Autodesk Fusion 360 part; units mm, degrees
note: some values were not read from the file. Chosen so that the rebuilt part matches the saved one: a side. Set by a fixed rule: which sketch regions a step uses.
(part 2 of 2)
sketch "Sketch13" plane through (0, 0, 19.74) normal (0, 0, -1) x (-1, 0, 0)
  line L0 (59.2047, 4.6574) -> (48.6047, 15.1574)
  line L1 (48.6047, -14.8158) -> (59.2047, -4.3158)
  arc A0 (-51.6422, 17.0699) -> (-55.1422, 13.5699) centre (-51.6422, 13.5699) ccw
  arc A1 (35.5416, -3.8292) -> (37.5416, -1.8292) centre (35.5416, -1.8292) ccw
  line L2 (47.9916, -8.3292) -> (47.9916, -12.3292)
  arc A2 (46.1416, -3.6792) -> (47.9916, -1.8292) centre (46.1416, -1.8292) ccw
  arc A3 (-47.6422, 7.7199) -> (-45.7922, 9.5699) centre (-47.6422, 9.5699) ccw
  line L3 (52.7416, 4.0208) -> (56.7416, 4.0208)
  line L4 (40.2916, -12.3292) -> (40.2916, -8.3292)
  line L5 (40.2916, -1.8292) -> (40.2916, 2.1708)
  arc A4 (-45.6422, -7.4301) -> (-47.6422, -5.4301) centre (-47.6422, -7.4301) ccw
  line L6 (39.6785, 15.1574) -> (29.0785, 4.6574)
  line L7 (58.5916, 2.1708) -> (58.5916, -1.8292)
  line L8 (40.2916, 8.6708) -> (40.2916, 12.6708)
  arc A5 (-47.6422, 7.5699) -> (-45.6422, 9.5699) centre (-47.6422, 9.5699) ccw
  arc A6 (46.1416, 6.8208) -> (47.9916, 8.6708) centre (46.1416, 8.6708) ccw
  line L9 (46.1416, 16.1708) -> (42.1416, 16.1708)
  arc A7 (42.1416, -6.4792) -> (40.2916, -8.3292) centre (42.1416, -8.3292) ccw
  line L10 (37.3916, 2.1708) -> (37.3916, -1.8292)
  arc A8 (42.1416, 4.0208) -> (40.2916, 2.1708) centre (42.1416, 2.1708) ccw
  arc A9 (-51.6422, -5.4301) -> (-53.6422, -7.4301) centre (-51.6422, -7.4301) ccw
  arc A10 (40.2916, 8.6708) -> (42.1416, 6.8208) centre (42.1416, 8.6708) ccw
  line L11 (46.1416, -15.8292) -> (48.451, -15.8292) construction
  line L12 (50.8916, -1.8292) -> (50.8916, 2.1708)
  arc A11 (29.5416, -1.8292) -> (31.5416, -3.8292) centre (31.5416, -1.8292) ccw
  line L13 (-45.6422, -7.4301) -> (-45.6422, -11.4301)
  line L14 (42.1416, -6.4792) -> (46.1416, -6.4792)
  arc A12 (60.2416, 2.1708) -> (56.7416, 5.6708) centre (56.7416, 2.1708) ccw
  arc A13 (37.5416, 2.1708) -> (35.5416, 4.1708) centre (35.5416, 2.1708) ccw
  arc A14 (58.5916, 2.1708) -> (56.7416, 4.0208) centre (56.7416, 2.1708) ccw
  line L15 (-45.6422, 13.5699) -> (-45.6422, 9.5699)
  arc A15 (42.1416, 14.5208) -> (40.2916, 12.6708) centre (42.1416, 12.6708) ccw
  arc A16 (50.8916, -1.8292) -> (52.7416, -3.6792) centre (52.7416, -1.8292) ccw
  line L16 (42.1416, 14.5208) -> (46.1416, 14.5208)
  line L17 (-47.6422, -13.4301) -> (-51.6422, -13.4301)
  arc A17 (40.2916, -1.8292) -> (42.1416, -3.6792) centre (42.1416, -1.8292) ccw
  line L18 (-47.6422, 7.5699) -> (-51.6422, 7.5699)
  line L19 (28.0416, 2.1708) -> (28.0416, -1.8292)
  line L20 (31.5416, 4.0208) -> (35.5416, 4.0208)
  line L21 (47.9916, 12.6708) -> (47.9916, 8.6708)
  line L22 (42.1416, 4.0208) -> (46.1416, 4.0208)
  line L23 (-53.6422, 9.5699) -> (-53.6422, 13.5699)
  arc A18 (47.9916, 2.1708) -> (46.1416, 4.0208) centre (46.1416, 2.1708) ccw
  arc A19 (49.6416, 12.6708) -> (46.1416, 16.1708) centre (46.1416, 12.6708) ccw
  line L24 (-51.6422, 15.5699) -> (-47.6422, 15.5699)
  arc A20 (28.0416, -1.8292) -> (31.5416, -5.3292) centre (31.5416, -1.8292) ccw
  line L25 (47.9916, 2.1708) -> (47.9916, -1.8292)
  arc A21 (46.1416, -15.8292) -> (49.6416, -12.3292) centre (46.1416, -12.3292) ccw
  arc A22 (52.7416, 4.0208) -> (50.8916, 2.1708) centre (52.7416, 2.1708) ccw
  arc A23 (-51.6422, 15.5699) -> (-53.6422, 13.5699) centre (-51.6422, 13.5699) ccw
  line L26 (46.1416, -3.6792) -> (42.1416, -3.6792)
  line L27 (-53.6422, -11.4301) -> (-53.6422, -7.4301)
  line L28 (56.7416, -3.6792) -> (52.7416, -3.6792)
  arc A24 (-45.7922, 13.5699) -> (-47.6422, 15.4199) centre (-47.6422, 13.5699) ccw
  arc A25 (-47.6422, -13.2801) -> (-45.7922, -11.4301) centre (-47.6422, -11.4301) ccw
  line L29 (29.0785, -4.3158) -> (39.6785, -14.8158)
  arc A26 (29.6916, -1.8292) -> (31.5416, -3.6792) centre (31.5416, -1.8292) ccw
  arc A27 (40.2916, -12.3292) -> (42.1416, -14.1792) centre (42.1416, -12.3292) ccw
  arc A28 (-44.1422, 13.5699) -> (-47.6422, 17.0699) centre (-47.6422, 13.5699) ccw
  arc A29 (38.6416, -12.3292) -> (42.1416, -15.8292) centre (42.1416, -12.3292) ccw
  line L30 (-45.7922, 13.5699) -> (-45.7922, 9.5699)
  line L31 (44.1416, -14.6745) -> (42.1416, -15.8292)
  line L32 (-51.6422, 17.0699) -> (-47.6422, 17.0699)
  line L33 (46.1416, -14.1792) -> (42.1416, -14.1792)
  arc A30 (-51.6422, -5.5801) -> (-53.4922, -7.4301) centre (-51.6422, -7.4301) ccw
  arc A31 (56.7416, -5.3292) -> (60.2416, -1.8292) centre (56.7416, -1.8292) ccw
  arc A32 (-51.6422, 15.4199) -> (-53.4922, 13.5699) centre (-51.6422, 13.5699) ccw
  line L34 (-55.1422, -11.4301) -> (-55.1422, 13.5699)
  line L35 (29.5416, -1.8292) -> (29.5416, 2.1708)
  arc A33 (31.5416, 4.0208) -> (29.6916, 2.1708) centre (31.5416, 2.1708) ccw
  arc A34 (-53.4922, -11.4301) -> (-51.6422, -13.2801) centre (-51.6422, -11.4301) ccw
  arc A35 (-53.4922, 9.5699) -> (-51.6422, 7.7199) centre (-51.6422, 9.5699) ccw
  line L36 (-47.6422, -14.9301) -> (-51.6422, -14.9301)
  line L37 (-53.4922, 9.5699) -> (-53.4922, 13.5699)
  line L38 (-44.1422, -11.4301) -> (-44.1422, 13.5699)
  line L39 (31.5416, 4.1708) -> (35.5416, 4.1708)
  arc A36 (-45.7922, -7.4301) -> (-47.6422, -5.5801) centre (-47.6422, -7.4301) ccw
  arc A37 (-47.6422, -14.9301) -> (-44.1422, -11.4301) centre (-47.6422, -11.4301) ccw
  arc A38 (35.5416, -3.6792) -> (37.3916, -1.8292) centre (35.5416, -1.8292) ccw
  line L40 (-45.7922, -7.4301) -> (-45.7922, -11.4301)
  line L41 (-51.6422, -5.5801) -> (-47.6422, -5.5801)
  line L42 (35.5416, -3.8292) -> (31.5416, -3.8292)
  line L43 (-47.6422, 7.7199) -> (-51.6422, 7.7199)
  line L44 (46.1416, -15.8292) -> (44.1416, -14.6745)
  arc A39 (47.9916, -8.3292) -> (46.1416, -6.4792) centre (46.1416, -8.3292) ccw
  arc A40 (31.5416, 5.6708) -> (28.0416, 2.1708) centre (31.5416, 2.1708) ccw
  line L45 (35.5416, -3.6792) -> (31.5416, -3.6792)
  line L46 (37.5416, 2.1708) -> (37.5416, -1.8292)
  arc A41 (56.7416, -3.6792) -> (58.5916, -1.8292) centre (56.7416, -1.8292) ccw
  line L47 (42.1416, -15.8292) -> (45.0396, -15.8292) construction
  arc A42 (-55.1422, -11.4301) -> (-51.6422, -14.9301) centre (-51.6422, -11.4301) ccw
  line L48 (42.1416, -15.8292) -> (46.1416, -15.8292)
  line L49 (-47.6422, -13.2801) -> (-51.6422, -13.2801)
  arc A43 (42.1416, 16.1708) -> (38.6416, 12.6708) centre (42.1416, 12.6708) ccw
  line L50 (46.1416, -3.8292) -> (42.1416, -3.8292)
  arc A44 (-45.6422, 13.5699) -> (-47.6422, 15.5699) centre (-47.6422, 13.5699) ccw
  line L51 (46.1416, 6.8208) -> (42.1416, 6.8208)
  line L52 (29.6916, -1.8292) -> (29.6916, 2.1708)
  arc A45 (46.1416, -14.1792) -> (47.9916, -12.3292) centre (46.1416, -12.3292) ccw
  line L53 (60.2416, -1.8292) -> (60.2416, 2.1708)
  line L54 (-51.6422, 15.4199) -> (-47.6422, 15.4199)
  line L55 (-53.4922, -11.4301) -> (-53.4922, -7.4301)
  arc A46 (37.3916, 2.1708) -> (35.5416, 4.0208) centre (35.5416, 2.1708) ccw
  arc A47 (31.5416, 4.1708) -> (29.5416, 2.1708) centre (31.5416, 2.1708) ccw
  arc A48 (-53.6422, -11.4301) -> (-51.6422, -13.4301) centre (-51.6422, -11.4301) ccw
  arc A49 (40.1416, -1.8292) -> (42.1416, -3.8292) centre (42.1416, -1.8292) ccw
  line L56 (46.1416, 6.6708) -> (42.1416, 6.6708)
  arc A50 (40.1416, -12.3292) -> (42.1416, -14.3292) centre (42.1416, -12.3292) ccw
  line L57 (48.1416, 2.1708) -> (48.1416, -1.8292)
  arc A51 (-53.6422, 9.5699) -> (-51.6422, 7.5699) centre (-51.6422, 9.5699) ccw
  arc A52 (46.1416, -3.8292) -> (48.1416, -1.8292) centre (46.1416, -1.8292) ccw
  line L58 (52.7416, 4.1708) -> (56.7416, 4.1708)
  arc A53 (40.1416, 8.6708) -> (42.1416, 6.6708) centre (42.1416, 8.6708) ccw
  arc A54 (42.1416, -6.3292) -> (40.1416, -8.3292) centre (42.1416, -8.3292) ccw
  arc A55 (47.9916, 12.6708) -> (46.1416, 14.5208) centre (46.1416, 12.6708) ccw
  arc A56 (56.7416, -3.8292) -> (58.7416, -1.8292) centre (56.7416, -1.8292) ccw
  line L59 (42.1416, -6.3292) -> (46.1416, -6.3292)
  line L60 (42.1416, 14.6708) -> (46.1416, 14.6708)
  line L61 (48.1416, 12.6708) -> (48.1416, 8.6708)
  arc A57 (58.7416, 2.1708) -> (56.7416, 4.1708) centre (56.7416, 2.1708) ccw
  line L62 (46.1416, -14.3292) -> (42.1416, -14.3292)
  line L63 (40.1416, -12.3292) -> (40.1416, -8.3292)
  arc A58 (42.1416, 14.6708) -> (40.1416, 12.6708) centre (42.1416, 12.6708) ccw
  line L64 (56.7416, -3.8292) -> (52.7416, -3.8292)
  arc A59 (-47.6422, -13.4301) -> (-45.6422, -11.4301) centre (-47.6422, -11.4301) ccw
  arc A60 (46.1416, -14.3292) -> (48.1416, -12.3292) centre (46.1416, -12.3292) ccw
  line L65 (50.7416, -1.8292) -> (50.7416, 2.1708)
  arc A61 (50.7416, -1.8292) -> (52.7416, -3.8292) centre (52.7416, -1.8292) ccw
  arc A62 (42.1416, 4.1708) -> (40.1416, 2.1708) centre (42.1416, 2.1708) ccw
  line L66 (40.1416, 8.6708) -> (40.1416, 12.6708)
  arc A63 (48.1416, -8.3292) -> (46.1416, -6.3292) centre (46.1416, -8.3292) ccw
  arc A64 (48.1416, 12.6708) -> (46.1416, 14.6708) centre (46.1416, 12.6708) ccw
  line L67 (48.1416, -8.3292) -> (48.1416, -12.3292)
  line L68 (40.1416, -1.8292) -> (40.1416, 2.1708)
  line L69 (42.1416, 4.1708) -> (46.1416, 4.1708)
  arc A65 (52.7416, 4.1708) -> (50.7416, 2.1708) centre (52.7416, 2.1708) ccw
  line L70 (-51.6422, -5.4301) -> (-47.6422, -5.4301)
  arc A66 (48.1416, 2.1708) -> (46.1416, 4.1708) centre (46.1416, 2.1708) ccw
  arc A67 (46.1416, 6.6708) -> (48.1416, 8.6708) centre (46.1416, 8.6708) ccw
  line L71 (58.7416, 2.1708) -> (58.7416, -1.8292)
  arc A68 (-47.6422, -2.9301) -> (-45.6422, -0.9301) centre (-47.6422, -0.9301) ccw
  arc A69 (-45.6422, 3.0699) -> (-47.6422, 5.0699) centre (-47.6422, 3.0699) ccw
  line L72 (-53.4922, -0.9301) -> (-53.4922, 3.0699)
  arc A70 (-47.6422, -2.7801) -> (-45.7922, -0.9301) centre (-47.6422, -0.9301) ccw
  line L73 (-45.7922, 3.0699) -> (-45.7922, -0.9301)
  line L74 (-45.6422, 3.0699) -> (-45.6422, -0.9301)
  line L75 (-51.6422, 5.0699) -> (-47.6422, 5.0699)
  arc A71 (-53.4922, -0.9301) -> (-51.6422, -2.7801) centre (-51.6422, -0.9301) ccw
  arc A72 (-51.6422, 4.9199) -> (-53.4922, 3.0699) centre (-51.6422, 3.0699) ccw
  line L76 (-47.6422, -2.9301) -> (-51.6422, -2.9301)
  arc A73 (-45.7922, 3.0699) -> (-47.6422, 4.9199) centre (-47.6422, 3.0699) ccw
  arc A74 (-51.6422, 5.0699) -> (-53.6422, 3.0699) centre (-51.6422, 3.0699) ccw
  line L77 (-47.6422, -2.7801) -> (-51.6422, -2.7801)
  line L78 (-51.6422, 4.9199) -> (-47.6422, 4.9199)
  line L79 (-53.6422, -0.9301) -> (-53.6422, 3.0699)
  arc A75 (-53.6422, -0.9301) -> (-51.6422, -2.9301) centre (-51.6422, -0.9301) ccw
  line L80 (-49.6422, -14.9301) -> (-49.6422, 17.0699) construction
  line L81 (-49.6422, -5.5801) -> (-49.6422, -4.1801) construction
  line L82 (-49.6422, 4.9199) -> (-49.6422, 6.3199) construction
  line L83 (-49.6422, 17.0699) -> (-49.6422, 16.2449) construction
  arc A76 (-55.1422, 8.8199) -> (-53.2922, 6.9699) centre (-53.2922, 8.8199) ccw
  arc A77 (-53.2922, -4.8301) -> (-55.1422, -6.6801) centre (-53.2922, -6.6801) ccw
  arc A78 (-53.2922, 5.6699) -> (-55.1422, 3.8199) centre (-53.2922, 3.8199) ccw
  arc A79 (-55.1422, -1.6801) -> (-53.2922, -3.5301) centre (-53.2922, -1.6801) ccw
  arc A80 (-49.6422, 5.6699) -> (-49.6422, 6.9699) centre (-49.6422, 6.3199) ccw
  line L84 (-49.6422, 6.9699) -> (-53.2922, 6.9699)
  line L85 (-53.2922, 5.6699) -> (-49.6422, 5.6699)
  arc A81 (-49.6422, -4.8301) -> (-49.6422, -3.5301) centre (-49.6422, -4.1801) ccw
  line L86 (-53.2922, -3.5301) -> (-49.6422, -3.5301)
  line L87 (-53.2922, -4.8301) -> (-49.6422, -4.8301)
  point P0 (42.95, -0.15)
  point P1 (0, -0.15)
  point P2 (-38.4431, -20.574)
  point P3 (-35.0431, -20.574)
  point P4 (23.3574, -20.574)
  point P5 (19.9574, -20.574)
  point P6 (-47.6422, -0.9301)
  point P7 (-51.6422, -0.9301)
  dimension "d137" = 0.15
  dimension "d138" = 0.15
  dimension "d139" = 0.15
  dimension "d140" = 0.15
  dimension "d141" = 0.15
  dimension "d142" = 0.15
  dimension "d144" = 0.15
  dimension "d145" = 1.5
  dimension "d146" = 1.5
  dimension "d147" = 1.5
  dimension "d148" = 1.5
  dimension "d149" = 1.5
  dimension "d150" = 1.5
  dimension "d151" = 1.5
  dimension "d152" = 1.5
  dimension "d153" = 1.5
  dimension "d154" = 1.5
  dimension "d155" = 150
  dimension "d156" = 0.15
  dimension "d185" = 1.4
  dimension "d186" = 1.4
  dimension "d190" = 0.825
  dimension "d193" = 0.65
  dimension "d194" = 0.65
  constraint coincident L1.start A21
  constraint coincident L1.end A31
  constraint tangent L1 A21
  constraint tangent L1 A31
  constraint coincident L0.start A12
  constraint coincident L0.end A19
  constraint coincident L6.start A43
  constraint coincident L6.end A40
  constraint coincident L29.start A20
  constraint coincident L29.end A29
  constraint tangent L0 A12
  constraint tangent L0 A19
  constraint tangent L6 A43
  constraint tangent L6 A40
  constraint tangent L29 A29
  constraint tangent A20 L29
  constraint tangent A21 L48
  constraint tangent A12 L53
  constraint tangent L9 A43
  constraint tangent L19 A20
  constraint tangent A0 L34
  constraint tangent A28 L38
  constraint horizontal L47
  constraint horizontal L11
  constraint midpoint L36 L80.start
  constraint midpoint L32 L80.end
  constraint perpendicular L32 L80
  constraint midpoint L41 L81.start
  constraint perpendicular L41 L81
  constraint midpoint L78 L82.start
  constraint perpendicular L75 L82
  constraint perpendicular L32 L83
  constraint coincident L80 A80.start
  constraint coincident L82.end A80.centre
  constraint tangent A76 L84
  constraint tangent A80 L85
  constraint coincident L80 A81.start
  constraint coincident L81.end A81.centre
  constraint tangent A81 L86
  constraint tangent A81 L87
  measures "d155" angle of L11 L44
  measures "d185" distance of L81.start L81.end
  measures "d186" distance of L82.start L82.end
  measures "d190" distance of L80.end L83.end
  measures "d193" radius of A80
  measures "d194" radius of A81
extrude "Extrude20" add sketch "Sketch13" along normal blind 0.2 separate body contours L0 L1 L6 L9 A12 L19 A19 A20 A21 L29 A29 L31 A31 L44 A40 A43 L53 | A0 A28 L32 L34 L36 L38 A37 A42 A76 A77 A78 A79 A80 L84 L85 A81 L86 L87 | A1 A11 A13 L35 L39 L42 L46 A47 | L2 L4 A7 L14 A27 L33 A39 A45 | A2 L5 A8 A17 L22 A18 L25 L26 | A3 A24 L30 A32 A35 L37 L43 L54 | L3 L7 L12 A14 A16 A22 L28 A41 | A4 A9 L13 L17 L27 A48 A59 L70 | L8 A6 A10 A15 L16 L21 L51 A55 | A5 L15 L18 L23 L24 A23 A44 A51 | L10 L20 A26 A33 A38 L45 L52 A46 | A25 A30 A34 A36 L40 L41 L49 L55 | L50 A49 L57 A52 A62 L68 L69 A66 | L56 A53 L60 L61 A58 L66 A64 A67 | A50 A54 L59 L62 L63 A60 A63 L67 | L58 A56 A57 L64 L65 A61 A65 L71 | A68 A69 L74 L75 L76 A74 L79 A75 | L72 A70 L73 A71 A72 A73 L77 L78 makes body 3 at (45.7739, 2.7408, 19.74) makes body 4 at (-50.6503, 1.7134, 19.74)
extrude "Extrude21" add sketch "Sketch13" against normal blind 4 contours L2 L4 A7 L14 A27 L33 A39 A45 | A2 L5 A8 A17 L22 A18 L25 L26 | A3 A24 L30 A32 A35 L37 L43 L54 | L3 L7 L12 A14 A16 A22 L28 A41 | L8 A6 A10 A15 L16 L21 L51 A55 | L10 L20 A26 A33 A38 L45 L52 A46 | A25 A30 A34 A36 L40 L41 L49 L55 | L72 A70 L73 A71 A72 A73 L77 L78 bodies 3 4
fillet "Fillet3" radius 1.25 64 edges at (46.3341, 14.8781, 23.74) (45.7922, 11.5699, 23.74) (46.3341, 8.2618, 23.74) (49.6422, 7.7199, 23.74) (52.9504, 8.2618, 23.74) (53.4922, 11.5699, 23.74) (52.9504, 14.8781, 23.74) (49.6422, 15.4199, 23.74) (45.7922, 1.0699, 23.74) (46.3341, -2.2382, 23.74) (49.6422, -2.7801, 23.74) (52.9504, -2.2382, 23.74) (53.4922, 1.0699, 23.74) (52.9504, 4.3781, 23.74) (49.6422, 4.9199, 23.74) (46.3341, 4.3781, 23.74) (45.7922, -9.4301, 23.74) (46.3341, -12.7382, 23.74) (49.6422, -13.2801, 23.74) (52.9504, -12.7382, 23.74) (53.4922, -9.4301, 23.74) (52.9504, -6.1219, 23.74) (49.6422, -5.5801, 23.74) (46.3341, -6.1219, 23.74) (-47.9916, 10.6708, 23.74) (-47.4497, 7.3627, 23.74) (-44.1416, 6.8208, 23.74) (-40.8334, 7.3627, 23.74) (-40.2916, 10.6708, 23.74) (-40.8334, 13.979, 23.74) (-44.1416, 14.5208, 23.74) (-47.4497, 13.979, 23.74) (-58.0497, 3.479, 23.74) (-58.5916, 0.1708, 23.74) (-58.0497, -3.1373, 23.74) (-54.7416, -3.6792, 23.74) (-51.4334, -3.1373, 23.74) (-50.8916, 0.1708, 23.74) (-51.4334, 3.479, 23.74) (-54.7416, 4.0208, 23.74) (-44.1416, -3.6792, 23.74) (-40.8334, -3.1373, 23.74) (-40.2916, 0.1708, 23.74) (-40.8334, 3.479, 23.74) (-44.1416, 4.0208, 23.74) (-47.4497, 3.479, 23.74) (-47.9916, 0.1708, 23.74) (-47.4497, -3.1373, 23.74) (-33.5416, -3.6792, 23.74) (-30.2334, -3.1373, 23.74) (-29.6916, 0.1708, 23.74) (-30.2334, 3.479, 23.74) (-33.5416, 4.0208, 23.74) (-36.8497, 3.479, 23.74) (-37.3916, 0.1708, 23.74) (-36.8497, -3.1373, 23.74) (-44.1416, -6.4792, 23.74) (-47.4497, -7.021, 23.74) (-47.9916, -10.3292, 23.74) (-47.4497, -13.6373, 23.74) (-44.1416, -14.1792, 23.74) (-40.8334, -13.6373, 23.74) (-40.2916, -10.3292, 23.74) (-40.8334, -7.021, 23.74) on bodies 3 4
sketch "Sketch14" plane through (0, 0, 15.25) normal (0, 0, 1) x (-1, 0, 0)
  line L0 (-16.3504, 12.3135) -> (-16.3504, 10.4179)
  line L1 (-16.3504, 10.4179) -> (-9.4158, 10.4179)
  line L2 (-9.4158, 10.4179) -> (-9.4158, 26.25)
  line L3 (-9.4158, 26.25) -> (-16.4158, 26.25)
  line L4 (-16.4158, 26.25) -> (-16.4158, 18.1418)
  line L5 (-16.4158, 18.1418) -> (-16.0557, 17.6179)
  line L6 (-16.0557, 17.6179) -> (-13.7656, 17.551)
  arc A0 (-13.7656, 12.3135) -> (-13.7656, 17.551) centre (-14.2529, 14.9323) ccw
  line L7 (-13.7656, 12.3135) -> (-16.3504, 12.3135)
  line L8 (-37.1008, 10.4179) -> (-37.1008, 12.3135)
  line L9 (-37.1008, 12.3135) -> (-39.6855, 12.3135)
  arc A1 (-39.6855, 17.551) -> (-39.6855, 12.3135) centre (-39.1982, 14.9323) ccw
  line L10 (-39.6855, 17.551) -> (-37.3955, 17.6179)
  line L11 (-37.3955, 17.6179) -> (-37.0353, 18.1418)
  line L12 (-37.0353, 18.1418) -> (-37.0353, 26.25)
  line L13 (-16.3504, 12.3135) -> (-37.1008, 12.3135)
  line L14 (-16.4158, 18.1418) -> (-16.4158, 26.1418)
  line L15 (-16.4158, 26.1418) -> (-37.0353, 26.1418)
  dimension "d163" = 8
  constraint coincident L0.start L7.end
  constraint coincident L8.end L9.start
  constraint coincident L4.end L5.start
  constraint perpendicular L3 L14
  constraint horizontal L15
  constraint coincident L12 L15.end
  measures "d163" distance of L4.end L14.end
extrude "Extrude22" add sketch "Sketch14" against normal blind 1 separate body contours L4 L5 L6 A0 L7 L9 A1 L10 L11 L12 L13 L14 L15 makes body 5
chamfer "Chamfer5" distance 1 distance2 0.5 1 edges at (1.1631, 9.3052, 0) measured on face at (29.052, 2.2266, 0) on bodies 1
